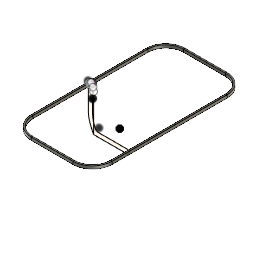
box_v3_o-ring_only (Autodesk Fusion 360 design; units mm, degrees)
Autodesk Fusion 360 part; units mm, degrees
sketch "Sketch1" plane through (0, 0, 0) normal (0, 1, 0) x (1, 0, 0)
  line L0 (-4, 12.7291) -> (-4, 24.6266)
  line L1 (0, 24.6266) -> (0, 12.7291)
  line L2 (-1.1892, 37.3052) -> (1, 42)
  line L3 (2.436, 35.6147) -> (2.4713, 35.6905)
  line L4 (35, 38) -> (6.0966, 38)
  line L5 (1, 6.3908) -> (1, 42)
  line L6 (1, 42) -> (35, 42)
  line L7 (35, 42) -> (35, 38)
  arc A0 (-1.1892, 37.3052) -> (-4, 24.6266) centre (26, 24.6266) ccw
  arc A1 (2.436, 35.6147) -> (0, 24.6266) centre (26, 24.6266) ccw
  arc A2 (6.0966, 38) -> (2.4713, 35.6905) centre (6.0966, 34) ccw
  line L8 (0, 12.7291) -> (0, 0)
  line L9 (0, 0) -> (-4, 0)
  line L10 (-4, 0) -> (-4, 12.7291)
  line L11 (-2.8767, 0) -> (-2.8767, -1.8)
  line L12 (-2.8767, 0) -> (-2.8767, 1.8)
  line L13 (-2.8767, -1.8) -> (-1.3767, 0)
  line L14 (-2.8767, 1.8) -> (-1.3767, 0)
  line L15 (-2.8767, 1.8) -> (-4.3767, 0)
  line L16 (-2.8767, -1.8) -> (-4.3767, 0)
  line L17 (-2.8767, -1.6438) -> (-4.2999, 0.064)
  line L18 (-2.8767, -1.6438) -> (-1.4535, 0.064)
  line L19 (-4, 0) -> (-6, 0)
  line L20 (-6, 0) -> (-6, 2.7)
  line L21 (-4, 1.5) -> (-4, 0)
  line L22 (-5.5915, 4.0695) -> (-4, 6.5)
  arc A3 (-5.5915, 4.0695) -> (-6, 2.7) centre (-3.5, 2.7) ccw
  line L23 (-1.3827, 0) -> (-4.3827, 0)
  line L24 (-4.3827, 0) -> (-1.3636, 0) construction
  line L25 (-3.8767, 0) -> (-1.8767, 0)
  line L26 (-1.8767, 0) -> (-1.8767, 3)
  line L27 (-1.8767, 3) -> (-3.8767, 3)
  line L28 (-3.8767, 3) -> (-3.8767, 0)
  line L29 (-1.8767, 3) -> (-1.9572, 0.6965)
  line L30 (-1.8767, 3) -> (0.4282, 3) construction
  line L31 (-3.8767, 3) -> (-3.7963, 0.6965)
  dimension "d5" = 4
  dimension "d6" = 30
  dimension "d7" = 26
  dimension "d8" = 4
  dimension "d9" = 1.8
  dimension "d10" = 1.8
  dimension "d11" = 1.5
  dimension "d12" = 1.5
  dimension "d13" = 0.1
  dimension "d30" = 4
  dimension "d33" = 4
  dimension "d36" = 5
  dimension "d38" = 35
  dimension "d60" = 25
  dimension "d113" = 2
  dimension "d115" = 2.5
  dimension "d126" = 6.5
  dimension "d334" = 4
  dimension "d335" = 38
  dimension "d486" = 1
  dimension "d487" = 1
  dimension "d488" = 3
  dimension "d489" = 2.8767
  dimension "d490" = 92
  dimension "d491" = 88
  measures "d6" radius of A0
  measures "d7" radius of A1
  measures "d8" radius of A2
  measures "d13" distance of L16
  measures "d33" distance of L8.end L10
  measures "d36" distance of L8.end L10
  measures "d60" angle of L2 L5
  measures "d113" distance of L20 L21
  measures "d115" radius of A3
  measures "d126" distance of L9
  measures "d335" distance of L8.end L4
  measures "d486" distance of L11 L28
  measures "d487" distance of L12 L26
  measures "d488" distance of L9 L27
  measures "d489" distance of L8.end L11
  measures "d490" angle of L29 L30
  measures "d491" angle of L30 L31
sketch "Sketch2" plane through (0, 0, 0) normal (0, 0, 1) x (1, 0, 0)
  line L0 (15, 70) -> (55, 70)
  line L1 (70, 55) -> (70, -55)
  line L2 (55, -70) -> (15, -70)
  line L3 (0, -55) -> (0, 55)
  arc A0 (15, 70) -> (0, 55) centre (15, 55) ccw
  arc A1 (70, 55) -> (55, 70) centre (55, 55) ccw
  arc A2 (55, -70) -> (70, -55) centre (55, -55) ccw
  arc A3 (0, -55) -> (15, -70) centre (15, -55) ccw
  dimension "d14" = 15
  dimension "d15" = 15
  dimension "d16" = 15
  dimension "d17" = 15
  dimension "d39" = 70
  dimension "d40" = 140
  measures "d14" radius of A0
  measures "d15" radius of A1
  measures "d16" radius of A2
  measures "d17" radius of A3
  measures "d39" distance of L1 L3
  measures "d40" distance of L0 L2
sketch "Sketch24" plane through (0, 0, 0) normal (0, 1, 0) x (1, 0, 0)
  line L0 (-1.8767, 3) -> (-3.8767, 3)
  line L1 (-3.7967, 3) -> (-3.6989, 0.2)
  line L2 (-4.3827, 0) -> (-1.3636, 0)
  line L3 (-3.6989, 0.2) -> (-2.0546, 0.2)
  line L4 (-2.0546, 0.2) -> (-1.9568, 3)
  line L5 (-1.9568, 3) -> (-3.7967, 3)
  line L6 (-3.8767, 3) -> (-3.7963, 0.6965)
  line L7 (-1.8767, 3) -> (-1.9572, 0.6965)
  arc A0 (-3.6989, 0.2) -> (-2.0546, 0.2) centre (-2.8767, 1.7053) ccw
  dimension "d493" = 0.08
  dimension "d494" = 0.08
  dimension "d495" = 2.8
  dimension "d538" = 1.7152
  measures "d493" distance of L4 L7
  measures "d494" distance of L1 L6
  measures "d495" distance of L3 L5
  measures "d538" radius of A0
sweep "Sweep4" add profiles "Sketch24" path "Sketch2" along A0 L0 A1 L1 A2 L2 A3 L3 section 1
equation "d5 = Twall"
equation "d6 = Rbase"
equation "d7 = Rbase - Twall"
equation "d14 = Rcorner"
equation "d15 = Rcorner"
equation "d16 = Rcorner"
equation "d17 = Rcorner"
equation "Twall = 4 mm"
equation "length = 140 mm"
equation "width = 70 mm"
equation "height = 38 mm"
equation "Rcorner = 15 mm"
equation "Rbase = 30 mm"
equation "d30 = Twall"
equation "d33 = Twall"
equation "d36 = base_inset"
equation "base_inset = 5 mm"
equation "d38 = width * 0.5"
equation "d39 = width"
equation "d40 = length"
equation "d60 = base_ang"
equation "base_ang = 25 deg"
equation "d334 = Twall"
equation "d335 = height"
equation "d495 = oringHeight"
equation "oringHeight = 2.8 mm"
named bodies: "O-Ring"
